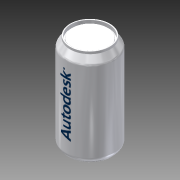
# Autodesk Inventor part: Can
Saved by Autodesk Inventor 2013 (Build 170138000, 138)
## iProperties
Created: 2008-06-06
Part Number: Can
Document SubType Name: Modeling
Designer: Phillip Dollan
Density: 1 g/cm^3
Material: Generic
Author: Phillip Dollan
Autodesk Inventor part; units mm, degrees
ref_plane "XZ Plane" through (0, 0, 0) normal (0, 1, 0) x (-1, 0, 0)
ref_plane "XY Plane" through (0, 0, 0) normal (0, 0, 1) x (1, 0, 0)
sketch "Sketch1" plane through (0, 0, 0) normal (0, 0, 1) x (1, 0, 0)
  line L0 (26.2727, -22.4856) -> (26.2727, 85.4644)
  line L1 (26.2727, 85.4644) -> (20.5713, 94.0487)
  line L2 (20.5713, 94.0487) -> (20.5713, 97.2237)
  line L3 (20.5713, 97.2237) -> (-5.4773, 97.2237)
  line L4 (-5.4773, 97.2237) -> (-5.4773, -43.5733) construction
  line L5 (-5.4773, 97.2237) -> (-5.4773, -26.7353)
  line L6 (26.2727, -22.4856) -> (22.2473, -25.1592)
  line L7 (22.2473, -25.1592) -> (22.2473, -26.7353)
  line L8 (22.2473, -26.7353) -> (-5.4773, -26.7353)
  dimension "d0" = 63.5
  dimension "d2" = 107.95
  dimension "d5" = 3.175
  constraints: 18 end point, 4 perpendicular, 2 parallel, 2 point on line, 1 vertical
  measures "d0" diameter of L0 L4
  measures "d2" distance of L0.start L0.end
  measures "d5" distance of L1.end L2.end
revolve "Revolution1" add sketch "Sketch1" angle 360 about axis through (-5.4773, 97.2237, 0) along (0, -1, 0)
ref_plane "Work Plane1" through (-5.4773, 95.6362, 0) normal (0, 0, 1) x (0, -1, 0)
sketch "Sketch2" plane through (-5.4773, 95.6362, 0) normal (0, 0, 1) x (0, -1, 0)
  line L0 (-1.5875, -26.0485) -> (-1.5875, 26.0485) projected
  line L1 (-1.5875, 26.0485) -> (1.5875, 26.0485) projected
  line L2 (-1.5875, 24.4987) -> (3.2582, 24.4987)
  line L3 (3.2582, 24.4987) -> (3.2582, 23.0371)
  line L4 (3.2582, 23.0371) -> (1.5875, 23.0371)
  line L5 (-76.977, 0) -> (450.7497, 0) construction
  line L6 (1.5875, 23.0371) -> (1.5875, 0) construction
  arc A0 (1.5875, 23.0371) -> (0.8353, 0) centre (375.3602, -0.6974) ccw
  line L7 (0.8353, 0) -> (-1.5875, 0)
  line L8 (-1.5875, 0) -> (-1.5875, 24.4987)
  constraints: 12 end point, 4 point on line, 2 parallel, 2 perpendicular, 2 point on circle, 1 centre point, 1 collinear, 1 midpoint
revolve "Revolution2" cut sketch "Sketch2" angle 360 about axis through (-5.4773, 95.6362, 0) along (0, -1, 0)
sketch "Sketch3" plane through (-5.4773, 95.6362, 0) normal (0, 0, 1) x (0, -1, 0)
  line L0 (122.3714, -27.7246) -> (122.3714, 27.7246) projected
  line L1 (122.3714, -27.7246) -> (122.3714, 27.7246) projected
  line L2 (120.7953, -27.7246) -> (120.7953, 27.7246) projected
  line L3 (118.1217, 31.75) -> (120.7953, 27.7246) projected
  line L4 (122.3714, 26.4057) -> (119.0201, 26.4057)
  line L5 (-26.3793, 0) -> (147.1632, 0) projected
  arc A0 (119.0201, 26.4057) -> (115.8621, 0) centre (224.5251, 0.3959) ccw
  line L6 (115.8621, 0) -> (122.3714, 0)
  line L7 (122.3714, 0) -> (122.3714, 26.4057)
  constraints: 6 end point, 3 point on line, 2 point on circle, 1 centre point, 1 collinear, 1 midpoint, 1 perpendicular
revolve "Revolution3" cut sketch "Sketch3" angle 360 about axis through (-5.4773, 95.6362, 0) along (0, -1, 0)
fillet "Fillet1" radius 6.35 2 edges at (-37.2273, 85.4644, 0) (-37.2273, -22.4856, 0)
fillet "Fillet2" radius 0.508 8 edges at (-28.5144, 94.0487, 0) (-31.5258, 94.0487, 0) (-33.2018, -25.1592, 0) (-31.8829, -23.384, 0) (-33.2018, -26.7353, 0) (-31.8829, -26.7353, 0) (-31.5258, 97.2237, 0) (-29.9759, 97.2237, 0)
ref_plane "Work Plane2" through (-5.4773, 95.6362, 39.6875) normal (0, 0, 1) x (0, -1, 0)
sketch "Sketch4" plane through (-5.4773, 95.6362, 39.6875) normal (0, 0, 1) x (0, -1, 0)
  line L0 (101.7128, -10.6178) -> (16.7903, -10.6178) construction
  line L1 (16.7903, -10.6178) -> (16.7903, 10.6178) construction
  line L2 (16.7903, 10.6178) -> (101.7128, 10.6178) construction
  line L3 (101.7128, 10.6178) -> (101.7128, -10.6178) construction
  line L4 (-1.0795, 26.0485) -> (-1.0795, -26.0485) projected
  line L5 (-1.0795, 0) -> (17.418, 0) construction
  point P0 (16.7903, 0)
  constraints: 2 end point, 2 horizontal, 2 midpoint, 1 horizontal alignment, 2 other
decal "Decal1"
body "Solid1"
